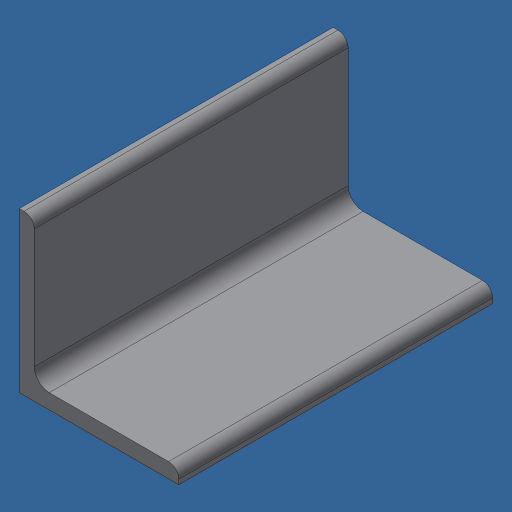
# Autodesk Inventor part: 3_ANGLE IRON, 2 X 2 X 0_25 THK
Saved by Autodesk Inventor 2024.3 (Build 283343000, 343)
## iProperties
Category: _
Manager: _
RuleStatus: InUse
Created: 2023-11-08
Part Number: 3_ANGLE IRON, 2 X 2 X 0_25 THK
Checked By: 0002612798
Engr Approved By: _
User Status: Work In Process
Material: Angle Iron
Description: 03_ANGLE IRON,TEMPLATE
Document SubType Name: Modeling
Mfg Approved By: Stephen.Oerton
Designer: -
Mass: 362.782 g
Surface Area: 207.607 cm^2
Volume: 46.1555 cm^3
Density: 7.86 g/cm^3
Appearance: Grey (Light)
ILogicPurgeVersion: 0.0.0.0
OnSaveVersion: 2.2.20.20
CN_MASS: 0.36
PTC_WM_ITERATION: 4
PTC_WM_ORGANIZATION_ID: CLWC
PTC_WM_LIFECYCLE: CLWC_CAD_LC
CN_SERVICEABLE: _
CL_runCount: 0
FinishProperty: ToBeSet
FIRST_DESCRIPTION: _
SECOND_DESCRIPTION: _
THIRD_DESCRIPTION: _
ModelCat: AngleIron
Length: 2.00" X 2.00" X 0.19" X 100.0 mm Lg
com.cntrline.rtcDoc: False
PROPOSAL_NUM: _
Subject: _
Author: -
Keywords: -
Revision Number: A
Autodesk Inventor part; units mm, degrees
ref_plane "YZ Plane" through (0, 0, 0) normal (1, 0, 0) x (0, 1, 0)
ref_plane "XZ Plane" through (0, 0, 0) normal (0, 1, 0) x (-1, 0, 0)
ref_plane "XY Plane" through (0, 0, 0) normal (0, 0, 1) x (1, 0, 0)
sketch "Sketch1" plane through (0, 0, 0) normal (0, 0, 1) x (1, 0, 0)
  line L0 (0, 0) -> (0, 50.8)
  line L1 (0, 50.8) -> (1.524, 50.8)
  line L2 (4.7625, 47.5615) -> (4.7625, 9.525)
  line L3 (0, 0) -> (50.8, 0)
  line L4 (50.8, 0) -> (50.8, 1.524)
  line L5 (47.5615, 4.7625) -> (9.525, 4.7625)
  arc A0 (4.7625, 9.525) -> (9.525, 4.7625) centre (9.525, 9.525) ccw
  arc A1 (4.7625, 47.5615) -> (1.524, 50.8) centre (1.524, 47.5615) ccw
  arc A2 (50.8, 1.524) -> (47.5615, 4.7625) centre (47.5615, 1.524) ccw
  dimension "d3" = 4.7625
  dimension "d7" = 3.2385
  dimension "d8" = 3.2385
  dimension "MidRad" = 4.7625
  constraints: 12 end point, 6 point on circle, 6 tangent, 5 parallel, 3 centre point, 1 coincident, 1 horizontal alignment, 1 perpendicular, 1 vertical, 1 vertical alignment
  measures "d3" distance between parallel lines of L5 L3
  measures "d7" radius of A1
  measures "d8" radius of A2
  measures "MidRad" radius of A0
extrude "Extrusion1" add sketch "Sketch1" along normal mid plane 100
